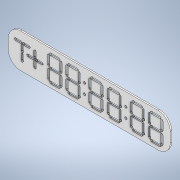
# Autodesk Inventor part: 7 Segment Clock
Saved by Autodesk Inventor 2021 (Build 250183000, 183)
## iProperties
Created: 2020-06-26
Part Number: 7 Segment Clock
Material: White
Document SubType Name: Modeling
Designer: dech3
Density: 1.188 g/cm^3
Appearance: Polycarbonate - Clear
Author: dech3
Autodesk Inventor part; units mm, degrees
(part 1 of 3)
ref_plane "YZ Plane" through (0, 0, 0) normal (1, 0, 0) x (0, 1, 0)
ref_plane "XZ Plane" through (0, 0, 0) normal (0, 1, 0) x (-1, 0, 0)
ref_plane "XY Plane" through (0, 0, 0) normal (0, 0, 1) x (1, 0, 0)
sketch "Single Segment" plane through (0, 0, 0) normal (0, 0, 1) x (1, 0, 0)
  arc A0 (128.9839, -2.0293) -> (129.691, -2.3222) centre (129.691, -1.3222) ccw
  arc A1 (129.691, 2.6778) -> (128.9839, 2.3849) centre (129.691, 1.6778) ccw
  line L0 (128.9839, -2.0293) -> (127.0768, -0.1222)
  line L1 (128.9839, 2.3849) -> (127.0768, 0.4778)
  line L2 (127.0768, 0.1778) -> (127.0768, -0.1222)
  line L3 (127.0768, 0.1778) -> (127.0768, 0.4778)
  line L4 (129.691, 2.6778) -> (146.4626, 2.6778)
  line L5 (146.4626, -2.3222) -> (129.691, -2.3222)
  arc A2 (147.1697, 2.3849) -> (146.4626, 2.6778) centre (146.4626, 1.6778) ccw
  line L6 (147.1697, 2.3849) -> (149.0768, 0.4778)
  line L7 (149.0768, 0.1778) -> (149.0768, 0.4778)
  line L8 (149.0768, 0.1778) -> (149.0768, -0.1222)
  arc A3 (146.4626, -2.3222) -> (147.1697, -2.0293) centre (146.4626, -1.3222) ccw
  line L9 (147.1697, -2.0293) -> (149.0768, -0.1222)
  point P0 (153.0768, 0)
  point P1 (129.2768, -2.3222)
  point P2 (129.2768, 2.6778)
  point P3 (146.8768, 2.6778)
  point P4 (146.8768, -2.3222)
  dimension "d105" = 2.2
  dimension "d108" = 2.2
  dimension "d111" = 2.2
  dimension "d112" = 2.2
  dimension "d113" = 2.2
  dimension "d114" = 2.2
  dimension "d115" = 2.2
  dimension "d116" = 1
  dimension "d117" = 5
  dimension "d121" = 2.2
  dimension "d122" = 2.2
  dimension "d126" = 135
  dimension "d127" = 22
  dimension "d128" = 135
  dimension "d129" = 2.5
  dimension "d348" = 5
  dimension "d349" = 22
  dimension "d350" = 2.2
  dimension "d352" = 0.3
  dimension "d353" = 0.3
  dimension "d358" = 0.3
  dimension "d359" = 0.3
  measures "d105" horizontal distance of point (129.277, -2.322) L0.end
  measures "d108" horizontal distance of L7.end point (146.877, 2.678)
  measures "d111" horizontal distance of point (129.277, 2.678) L3.end
  measures "d112" horizontal distance of L9.end point (146.877, -2.322)
  measures "d113" horizontal distance of L9.end point (146.877, -2.322)
  measures "d114" horizontal distance of point (129.277, 2.678) L3.end
  measures "d115" horizontal distance of point (129.277, -2.322) L0.end
  measures "d116" radius of A1
  measures "d117" distance of point (146.877, -2.322) point (146.877, 2.678)
  measures "d121" horizontal distance of L7.end point (146.877, 2.678)
  measures "d122" horizontal distance of point (146.877, -2.322) L8.start
  measures "d126" angle of L5 L9
  measures "d127" horizontal distance of L9.end L3.start
  measures "d128" angle of L4 L6
  measures "d129" vertical distance of L8.start point (146.877, -2.322)
  measures "d348" distance between parallel lines of L5 L4
  measures "d349" distance of L3.start L8.start
  measures "d350" horizontal distance of point (129.277, 2.678) L3.start
  measures "d352" distance of L8.start L7.end
  measures "d353" distance of L9.end L8.start
  measures "d358" distance of L3.end L3.start
  measures "d359" distance of L0.end L3.start
sketch "7 Segment Digit" plane through (0, 0, 0) normal (0, 0, 1) x (1, 0, 0)
  arc A0 (215.9071, -11.0293) -> (216.6142, -11.3222) centre (216.6142, -10.3222) ccw
  arc A1 (216.6142, -6.3222) -> (215.9071, -6.6151) centre (216.6142, -7.3222) ccw
  line L0 (215.9071, -11.0293) -> (214, -9.1222)
  line L1 (215.9071, -6.6151) -> (214, -8.5222)
  line L2 (214, -8.8222) -> (214, -9.1222)
  line L3 (214, -8.8222) -> (214, -8.5222)
  line L4 (216.6142, -6.3222) -> (233.3858, -6.3222)
  line L5 (233.3858, -11.3222) -> (216.6142, -11.3222)
  arc A2 (234.0929, -6.6151) -> (233.3858, -6.3222) centre (233.3858, -7.3222) ccw
  line L6 (234.0929, -6.6151) -> (236, -8.5222)
  line L7 (236, -8.8222) -> (236, -8.5222)
  line L8 (236, -8.8222) -> (236, -9.1222)
  arc A3 (233.3858, -11.3222) -> (234.0929, -11.0293) centre (233.3858, -10.3222) ccw
  line L9 (234.0929, -11.0293) -> (236, -9.1222)
  arc A4 (215.9071, -35.8293) -> (216.6142, -36.1222) centre (216.6142, -35.1222) ccw
  arc A5 (216.6142, -31.1222) -> (215.9071, -31.4151) centre (216.6142, -32.1222) ccw
  line L10 (215.9071, -35.8293) -> (214, -33.9222)
  line L11 (215.9071, -31.4151) -> (214, -33.3222)
  line L12 (214, -33.6222) -> (214, -33.9222)
  line L13 (214, -33.6222) -> (214, -33.3222)
  line L14 (216.6142, -31.1222) -> (233.3858, -31.1222)
  line L15 (233.3858, -36.1222) -> (216.6142, -36.1222)
  arc A6 (234.0929, -31.4151) -> (233.3858, -31.1222) centre (233.3858, -32.1222) ccw
  line L16 (234.0929, -31.4151) -> (236, -33.3222)
  line L17 (236, -33.6222) -> (236, -33.3222)
  line L18 (236, -33.6222) -> (236, -33.9222)
  arc A7 (233.3858, -36.1222) -> (234.0929, -35.8293) centre (233.3858, -35.1222) ccw
  line L19 (234.0929, -35.8293) -> (236, -33.9222)
  arc A8 (214.8071, -30.3151) -> (215.1, -29.608) centre (214.1, -29.608) ccw
  arc A9 (210.1, -29.608) -> (210.3929, -30.3151) centre (211.1, -29.608) ccw
  line L20 (214.8071, -30.3151) -> (212.9, -32.2222)
  line L21 (210.3929, -30.3151) -> (212.3, -32.2222)
  line L22 (212.6, -32.2222) -> (212.9, -32.2222)
  line L23 (212.6, -32.2222) -> (212.3, -32.2222)
  line L24 (210.1, -29.608) -> (210.1, -12.8364)
  line L25 (215.1, -12.8364) -> (215.1, -29.608)
  arc A10 (210.3929, -12.1293) -> (210.1, -12.8364) centre (211.1, -12.8364) ccw
  line L26 (210.3929, -12.1293) -> (212.3, -10.2222)
  line L27 (212.6, -10.2222) -> (212.3, -10.2222)
  line L28 (212.6, -10.2222) -> (212.9, -10.2222)
  arc A11 (215.1, -12.8364) -> (214.8071, -12.1293) centre (214.1, -12.8364) ccw
  line L29 (214.8071, -12.1293) -> (212.9, -10.2222)
  arc A12 (214.8071, -55.1151) -> (215.1, -54.408) centre (214.1, -54.408) ccw
  arc A13 (210.1, -54.408) -> (210.3929, -55.1151) centre (211.1, -54.408) ccw
  line L30 (214.8071, -55.1151) -> (212.9, -57.0222)
  line L31 (210.3929, -55.1151) -> (212.3, -57.0222)
  line L32 (212.6, -57.0222) -> (212.9, -57.0222)
  line L33 (212.6, -57.0222) -> (212.3, -57.0222)
  line L34 (210.1, -54.408) -> (210.1, -37.6364)
  line L35 (215.1, -37.6364) -> (215.1, -54.408)
  arc A14 (210.3929, -36.9293) -> (210.1, -37.6364) centre (211.1, -37.6364) ccw
  line L36 (210.3929, -36.9293) -> (212.3, -35.0222)
  line L37 (212.6, -35.0222) -> (212.3, -35.0222)
  line L38 (212.6, -35.0222) -> (212.9, -35.0222)
  arc A15 (215.1, -37.6364) -> (214.8071, -36.9293) centre (214.1, -37.6364) ccw
  line L39 (214.8071, -36.9293) -> (212.9, -35.0222)
  arc A16 (239.6071, -30.3151) -> (239.9, -29.608) centre (238.9, -29.608) ccw
  arc A17 (234.9, -29.608) -> (235.1929, -30.3151) centre (235.9, -29.608) ccw
  line L40 (239.6071, -30.3151) -> (237.7, -32.2222)
  line L41 (235.1929, -30.3151) -> (237.1, -32.2222)
  line L42 (237.4, -32.2222) -> (237.7, -32.2222)
  line L43 (237.4, -32.2222) -> (237.1, -32.2222)
  line L44 (234.9, -29.608) -> (234.9, -12.8364)
  line L45 (239.9, -12.8364) -> (239.9, -29.608)
  arc A18 (235.1929, -12.1293) -> (234.9, -12.8364) centre (235.9, -12.8364) ccw
  line L46 (235.1929, -12.1293) -> (237.1, -10.2222)
  line L47 (237.4, -10.2222) -> (237.1, -10.2222)
  line L48 (237.4, -10.2222) -> (237.7, -10.2222)
  arc A19 (239.9, -12.8364) -> (239.6071, -12.1293) centre (238.9, -12.8364) ccw
  line L49 (239.6071, -12.1293) -> (237.7, -10.2222)
  arc A20 (239.6071, -55.1151) -> (239.9, -54.408) centre (238.9, -54.408) ccw
  arc A21 (234.9, -54.408) -> (235.1929, -55.1151) centre (235.9, -54.408) ccw
  line L50 (239.6071, -55.1151) -> (237.7, -57.0222)
  line L51 (235.1929, -55.1151) -> (237.1, -57.0222)
  line L52 (237.4, -57.0222) -> (237.7, -57.0222)
  line L53 (237.4, -57.0222) -> (237.1, -57.0222)
  line L54 (234.9, -54.408) -> (234.9, -37.6364)
  line L55 (239.9, -37.6364) -> (239.9, -54.408)
  arc A22 (235.1929, -36.9293) -> (234.9, -37.6364) centre (235.9, -37.6364) ccw
  line L56 (235.1929, -36.9293) -> (237.1, -35.0222)
  line L57 (237.4, -35.0222) -> (237.1, -35.0222)
  line L58 (237.4, -35.0222) -> (237.7, -35.0222)
  arc A23 (239.9, -37.6364) -> (239.6071, -36.9293) centre (238.9, -37.6364) ccw
  line L59 (239.6071, -36.9293) -> (237.7, -35.0222)
  arc A24 (215.9071, -60.6293) -> (216.6142, -60.9222) centre (216.6142, -59.9222) ccw
  arc A25 (216.6142, -55.9222) -> (215.9071, -56.2151) centre (216.6142, -56.9222) ccw
  line L60 (215.9071, -60.6293) -> (214, -58.7222)
  line L61 (215.9071, -56.2151) -> (214, -58.1222)
  line L62 (214, -58.4222) -> (214, -58.7222)
  line L63 (214, -58.4222) -> (214, -58.1222)
  line L64 (216.6142, -55.9222) -> (233.3858, -55.9222)
  line L65 (233.3858, -60.9222) -> (216.6142, -60.9222)
  arc A26 (234.0929, -56.2151) -> (233.3858, -55.9222) centre (233.3858, -56.9222) ccw
  line L66 (234.0929, -56.2151) -> (236, -58.1222)
  line L67 (236, -58.4222) -> (236, -58.1222)
  line L68 (236, -58.4222) -> (236, -58.7222)
  arc A27 (233.3858, -60.9222) -> (234.0929, -60.6293) centre (233.3858, -59.9222) ccw
  line L69 (234.0929, -60.6293) -> (236, -58.7222)
  point P0 (239.8857, -4.9143)
  dimension "d131" = 1.1
  dimension "d132" = 1.1
  dimension "d137" = 1.1
  dimension "d138" = 1.1
  dimension "d139" = 1.1
  dimension "d140" = 1.1
  dimension "d141" = 1.1
  dimension "d142" = 1.1
  dimension "d143" = 1.1
  dimension "d144" = 1.1
  dimension "d145" = 1.1
  dimension "d146" = 1.1
  dimension "d150" = 1.1
  dimension "d151" = 1.1
  dimension "d152" = 1.1
  dimension "d153" = 1.1
sketch "Slanted Segment Large" plane through (0, 0, 0) normal (0, 0, 1) x (1, 0, 0)
  line L0 (-252.8296, -124.6537) -> (-254.4296, -124.6537)
  line L1 (-254.4296, -124.6537) -> (-257.6296, -127.8537)
  line L2 (-257.6296, -127.8537) -> (-261.6917, -184.8537)
  line L3 (-253.6917, -184.8537) -> (-249.6296, -127.8537)
  line L4 (-249.6296, -127.8537) -> (-252.8296, -124.6537)
  line L5 (-261.6917, -184.8537) -> (-258.4917, -188.0537)
  line L6 (-258.4917, -188.0537) -> (-256.8917, -188.0537)
  line L7 (-256.8917, -188.0537) -> (-253.6917, -184.8537)
  point P0 (-253.3255, -154.094)
  point P1 (-253.6296, -124.6537)
  dimension "d294" = 3.2
  dimension "d295" = 3.2
  dimension "d296" = 8
  dimension "d297" = 3.2
  dimension "d298" = 3.2
  dimension "d299" = 57
  dimension "d304" = 3.2
  dimension "d305" = 3.2
  dimension "d306" = 3.2
  dimension "d307" = 3.2
  measures "d294" horizontal distance of L0.end L1.end
  measures "d295" horizontal distance of L3.end L0.start
  measures "d296" distance of L3.end L1.end
  measures "d297" horizontal distance of L3.end L0.start
  measures "d298" horizontal distance of L0.end L1.end
  measures "d299" vertical distance of L3.end L3.start
  measures "d304" horizontal distance of L5.end L2.end
  measures "d305" horizontal distance of L3.start L6.end
  measures "d306" horizontal distance of L2.end L5.end
  measures "d307" horizontal distance of L3.start L6.end
sketch "+ sign" plane through (0, 0, 0) normal (0, 0, 1) x (1, 0, 0)
  arc A0 (1.761, -2.8041) -> (2.4681, -3.097) centre (2.4681, -2.097) ccw
  arc A1 (2.4681, 1.903) -> (1.761, 1.6102) centre (2.4681, 0.903) ccw
  line L0 (1.761, -2.8041) -> (-0.1461, -0.897)
  line L1 (-0.1461, -0.597) -> (-0.1461, -0.297)
  line L2 (-0.1461, -0.597) -> (-0.1461, -0.897)
  line L3 (1.761, 1.6102) -> (-0.1461, -0.297)
  line L4 (2.4681, 1.903) -> (13.2397, 1.903)
  line L5 (13.2397, -3.097) -> (2.4681, -3.097)
  arc A2 (13.9468, 1.6102) -> (13.2397, 1.903) centre (13.2397, 0.903) ccw
  arc A3 (13.2397, -3.097) -> (13.9468, -2.8041) centre (13.2397, -2.097) ccw
  line L6 (13.9468, -2.8041) -> (15.8539, -0.897)
  line L7 (15.8539, -0.597) -> (15.8539, -0.897)
  line L8 (15.8539, -0.597) -> (15.8539, -0.297)
  line L9 (13.9468, 1.6102) -> (15.8539, -0.297)
  arc A4 (1.061, 2.3102) -> (1.3539, 3.0173) centre (0.3539, 3.0173) ccw
  arc A5 (-3.6461, 3.0173) -> (-3.3532, 2.3102) centre (-2.6461, 3.0173) ccw
  line L10 (1.061, 2.3102) -> (-0.8461, 0.403)
  line L11 (-1.1461, 0.403) -> (-1.4461, 0.403)
  line L12 (-1.1461, 0.403) -> (-0.8461, 0.403)
  line L13 (-3.3532, 2.3102) -> (-1.4461, 0.403)
  line L14 (-3.6461, 3.0173) -> (-3.6461, 13.7888)
  line L15 (1.3539, 13.7888) -> (1.3539, 3.0173)
  arc A6 (-3.3532, 14.4959) -> (-3.6461, 13.7888) centre (-2.6461, 13.7888) ccw
  arc A7 (1.3539, 13.7888) -> (1.061, 14.4959) centre (0.3539, 13.7888) ccw
  line L16 (1.061, 14.4959) -> (-0.8461, 16.403)
  line L17 (-1.1461, 16.403) -> (-0.8461, 16.403)
  line L18 (-1.1461, 16.403) -> (-1.4461, 16.403)
  line L19 (-3.3532, 14.4959) -> (-1.4461, 16.403)
  arc A8 (-16.239, -2.8041) -> (-15.5319, -3.097) centre (-15.5319, -2.097) ccw
  arc A9 (-15.5319, 1.903) -> (-16.239, 1.6102) centre (-15.5319, 0.903) ccw
  line L20 (-16.239, -2.8041) -> (-18.1461, -0.897)
  line L21 (-18.1461, -0.597) -> (-18.1461, -0.297)
  line L22 (-18.1461, -0.597) -> (-18.1461, -0.897)
  line L23 (-16.239, 1.6102) -> (-18.1461, -0.297)
  line L24 (-15.5319, 1.903) -> (-4.7603, 1.903)
  line L25 (-4.7603, -3.097) -> (-15.5319, -3.097)
  arc A10 (-4.0532, 1.6102) -> (-4.7603, 1.903) centre (-4.7603, 0.903) ccw
  arc A11 (-4.7603, -3.097) -> (-4.0532, -2.8041) centre (-4.7603, -2.097) ccw
  line L26 (-4.0532, -2.8041) -> (-2.1461, -0.897)
  line L27 (-2.1461, -0.597) -> (-2.1461, -0.897)
  line L28 (-2.1461, -0.597) -> (-2.1461, -0.297)
  line L29 (-4.0532, 1.6102) -> (-2.1461, -0.297)
  arc A12 (1.061, -15.6898) -> (1.3539, -14.9827) centre (0.3539, -14.9827) ccw
  arc A13 (-3.6461, -14.9827) -> (-3.3532, -15.6898) centre (-2.6461, -14.9827) ccw
  line L30 (1.061, -15.6898) -> (-0.8461, -17.597)
  line L31 (-1.1461, -17.597) -> (-1.4461, -17.597)
  line L32 (-1.1461, -17.597) -> (-0.8461, -17.597)
  line L33 (-3.3532, -15.6898) -> (-1.4461, -17.597)
  line L34 (-3.6461, -14.9827) -> (-3.6461, -4.2112)
  line L35 (1.3539, -4.2112) -> (1.3539, -14.9827)
  arc A14 (-3.3532, -3.5041) -> (-3.6461, -4.2112) centre (-2.6461, -4.2112) ccw
  arc A15 (1.3539, -4.2112) -> (1.061, -3.5041) centre (0.3539, -4.2112) ccw
  line L36 (1.061, -3.5041) -> (-0.8461, -1.597)
  line L37 (-1.1461, -1.597) -> (-0.8461, -1.597)
  line L38 (-1.1461, -1.597) -> (-1.4461, -1.597)
  line L39 (-3.3532, -3.5041) -> (-1.4461, -1.597)
  point P0 (-225.4266, -6.7349)
  dimension "d496" = 2
  dimension "d497" = 2
  dimension "d501" = 1
  dimension "d502" = 1
  dimension "d503" = 0
  dimension "d504" = 0
  dimension "d505" = 0.99
  dimension "d506" = 0.99
  dimension "d507" = 0.99
  dimension "d508" = 0.99
sketch "Dot" plane through (0, 0, 0) normal (0, 0, 1) x (1, 0, 0)
  line L0 (-36.1663, 28.3091) -> (-35.1663, 28.3091)
  line L1 (-35.1663, 28.3091) -> (-33.1663, 26.3091)
  line L2 (-33.1663, 26.3091) -> (-33.1663, 25.3091)
  line L3 (-33.1663, 25.3091) -> (-35.1663, 23.3091)
  line L4 (-35.1663, 23.3091) -> (-36.1663, 23.3091)
  line L5 (-36.1663, 23.3091) -> (-38.1663, 25.3091)
  line L6 (-38.1663, 25.3091) -> (-38.1663, 26.3091)
  line L7 (-38.1663, 26.3091) -> (-36.1663, 28.3091)
  point P0 (-33.9663, 25.3091)
  dimension "d311" = 2
  dimension "d312" = 2
  dimension "d314" = 2
  dimension "d315" = 2
  dimension "d316" = 2
  dimension "d317" = 2
  dimension "d318" = 2
  dimension "d319" = 2
  dimension "d320" = 1
  dimension "d321" = 1
  dimension "d322" = 1
  dimension "d323" = 1
  dimension "d360" = 5
  dimension "d361" = 5
  measures "d311" horizontal distance of L1.end L0.end
  measures "d312" horizontal distance of L0.start L6.end
  measures "d314" horizontal distance of L0.start L6.end
  measures "d315" horizontal distance of L1.end L0.end
  measures "d316" horizontal distance of L4.end L5.end
  measures "d317" horizontal distance of L2.end L3.end
  measures "d318" horizontal distance of L2.end L3.end
  measures "d319" horizontal distance of L5.end L4.end
  measures "d320" distance of L1.end L2.end
  measures "d321" distance of L0.end L0.start
  measures "d322" distance of L3.end L4.end
  measures "d323" distance of L6.end L5.end
  measures "d360" distance between parallel lines of L4 L0
  measures "d361" distance between parallel lines of L2 L6
sketch "Clock Face with T +-" plane through (0, 0, 0) normal (0, 0, 1) x (1, 0, 0)
  arc A0 (53.0672, 19.3353) -> (53.7743, 19.0424) centre (53.7743, 20.0424) ccw
  arc A1 (53.7743, 24.0424) -> (53.0672, 23.7495) centre (53.7743, 23.0424) ccw
  line L0 (53.0672, 19.3353) -> (51.1601, 21.2424)
  line L1 (53.0672, 23.7495) -> (51.1601, 21.8424)
  line L2 (51.1601, 21.5424) -> (51.1601, 21.2424)
  line L3 (51.1601, 21.5424) -> (51.1601, 21.8424)
  line L4 (53.7743, 24.0424) -> (70.5459, 24.0424)
  line L5 (70.5459, 19.0424) -> (53.7743, 19.0424)
  arc A2 (71.253, 23.7495) -> (70.5459, 24.0424) centre (70.5459, 23.0424) ccw
  line L6 (71.253, 23.7495) -> (73.1601, 21.8424)
  line L7 (73.1601, 21.5424) -> (73.1601, 21.8424)
  line L8 (73.1601, 21.5424) -> (73.1601, 21.2424)
  arc A3 (70.5459, 19.0424) -> (71.253, 19.3353) centre (70.5459, 20.0424) ccw
  line L9 (71.253, 19.3353) -> (73.1601, 21.2424)
  arc A4 (53.0672, -5.4647) -> (53.7743, -5.7576) centre (53.7743, -4.7576) ccw
  arc A5 (53.7743, -0.7576) -> (53.0672, -1.0505) centre (53.7743, -1.7576) ccw
  line L10 (53.0672, -5.4647) -> (51.1601, -3.5576)
  line L11 (53.0672, -1.0505) -> (51.1601, -2.9576)
  line L12 (51.1601, -3.2576) -> (51.1601, -3.5576)
  line L13 (51.1601, -3.2576) -> (51.1601, -2.9576)
  line L14 (53.7743, -0.7576) -> (70.5459, -0.7576)
  line L15 (70.5459, -5.7576) -> (53.7743, -5.7576)
  arc A6 (71.253, -1.0505) -> (70.5459, -0.7576) centre (70.5459, -1.7576) ccw
  line L16 (71.253, -1.0505) -> (73.1601, -2.9576)
  line L17 (73.1601, -3.2576) -> (73.1601, -2.9576)
  line L18 (73.1601, -3.2576) -> (73.1601, -3.5576)
  arc A7 (70.5459, -5.7576) -> (71.253, -5.4647) centre (70.5459, -4.7576) ccw
  line L19 (71.253, -5.4647) -> (73.1601, -3.5576)
  arc A8 (51.9672, 0.0495) -> (52.2601, 0.7566) centre (51.2601, 0.7566) ccw
  arc A9 (47.2601, 0.7566) -> (47.553, 0.0495) centre (48.2601, 0.7566) ccw
  line L20 (51.9672, 0.0495) -> (50.0601, -1.8576)
  line L21 (47.553, 0.0495) -> (49.4601, -1.8576)
  line L22 (49.7601, -1.8576) -> (50.0601, -1.8576)
  line L23 (49.7601, -1.8576) -> (49.4601, -1.8576)
  line L24 (47.2601, 0.7566) -> (47.2601, 17.5282)
  line L25 (52.2601, 17.5282) -> (52.2601, 0.7566)
  arc A10 (47.553, 18.2353) -> (47.2601, 17.5282) centre (48.2601, 17.5282) ccw
  line L26 (47.553, 18.2353) -> (49.4601, 20.1424)
  line L27 (49.7601, 20.1424) -> (49.4601, 20.1424)
  line L28 (49.7601, 20.1424) -> (50.0601, 20.1424)
  arc A11 (52.2601, 17.5282) -> (51.9672, 18.2353) centre (51.2601, 17.5282) ccw
  line L29 (51.9672, 18.2353) -> (50.0601, 20.1424)
  arc A12 (51.9672, -24.7505) -> (52.2601, -24.0434) centre (51.2601, -24.0434) ccw
  arc A13 (47.2601, -24.0434) -> (47.553, -24.7505) centre (48.2601, -24.0434) ccw
  line L30 (51.9672, -24.7505) -> (50.0601, -26.6576)
  line L31 (47.553, -24.7505) -> (49.4601, -26.6576)
  line L32 (49.7601, -26.6576) -> (50.0601, -26.6576)
  line L33 (49.7601, -26.6576) -> (49.4601, -26.6576)
  line L34 (47.2601, -24.0434) -> (47.2601, -7.2718)
  line L35 (52.2601, -7.2718) -> (52.2601, -24.0434)
  arc A14 (47.553, -6.5647) -> (47.2601, -7.2718) centre (48.2601, -7.2718) ccw
  line L36 (47.553, -6.5647) -> (49.4601, -4.6576)
  line L37 (49.7601, -4.6576) -> (49.4601, -4.6576)
  line L38 (49.7601, -4.6576) -> (50.0601, -4.6576)
  arc A15 (52.2601, -7.2718) -> (51.9672, -6.5647) centre (51.2601, -7.2718) ccw
  line L39 (51.9672, -6.5647) -> (50.0601, -4.6576)
  arc A16 (76.7672, 0.0495) -> (77.0601, 0.7566) centre (76.0601, 0.7566) ccw
  arc A17 (72.0601, 0.7566) -> (72.353, 0.0495) centre (73.0601, 0.7566) ccw
  line L40 (76.7672, 0.0495) -> (74.8601, -1.8576)
  line L41 (72.353, 0.0495) -> (74.2601, -1.8576)
  line L42 (74.5601, -1.8576) -> (74.8601, -1.8576)
  line L43 (74.5601, -1.8576) -> (74.2601, -1.8576)
  line L44 (72.0601, 0.7566) -> (72.0601, 17.5282)
  line L45 (77.0601, 17.5282) -> (77.0601, 0.7566)
  arc A18 (72.353, 18.2353) -> (72.0601, 17.5282) centre (73.0601, 17.5282) ccw
  line L46 (72.353, 18.2353) -> (74.2601, 20.1424)
  line L47 (74.5601, 20.1424) -> (74.2601, 20.1424)
  line L48 (74.5601, 20.1424) -> (74.8601, 20.1424)
  arc A19 (77.0601, 17.5282) -> (76.7672, 18.2353) centre (76.0601, 17.5282) ccw
  line L49 (76.7672, 18.2353) -> (74.8601, 20.1424)
  arc A20 (76.7672, -24.7505) -> (77.0601, -24.0434) centre (76.0601, -24.0434) ccw
  arc A21 (72.0601, -24.0434) -> (72.353, -24.7505) centre (73.0601, -24.0434) ccw
  line L50 (76.7672, -24.7505) -> (74.8601, -26.6576)
  line L51 (72.353, -24.7505) -> (74.2601, -26.6576)
  line L52 (74.5601, -26.6576) -> (74.8601, -26.6576)
  line L53 (74.5601, -26.6576) -> (74.2601, -26.6576)
  line L54 (72.0601, -24.0434) -> (72.0601, -7.2718)
  line L55 (77.0601, -7.2718) -> (77.0601, -24.0434)
  arc A22 (72.353, -6.5647) -> (72.0601, -7.2718) centre (73.0601, -7.2718) ccw
  line L56 (72.353, -6.5647) -> (74.2601, -4.6576)
  line L57 (74.5601, -4.6576) -> (74.2601, -4.6576)
  line L58 (74.5601, -4.6576) -> (74.8601, -4.6576)
  arc A23 (77.0601, -7.2718) -> (76.7672, -6.5647) centre (76.0601, -7.2718) ccw
  line L59 (76.7672, -6.5647) -> (74.8601, -4.6576)
  arc A24 (53.0672, -30.2647) -> (53.7743, -30.5576) centre (53.7743, -29.5576) ccw
  arc A25 (53.7743, -25.5576) -> (53.0672, -25.8505) centre (53.7743, -26.5576) ccw
  line L60 (53.0672, -30.2647) -> (51.1601, -28.3576)
  line L61 (53.0672, -25.8505) -> (51.1601, -27.7576)
  line L62 (51.1601, -28.0576) -> (51.1601, -28.3576)
  line L63 (51.1601, -28.0576) -> (51.1601, -27.7576)
  line L64 (53.7743, -25.5576) -> (70.5459, -25.5576)
  line L65 (70.5459, -30.5576) -> (53.7743, -30.5576)
  arc A26 (71.253, -25.8505) -> (70.5459, -25.5576) centre (70.5459, -26.5576) ccw
  line L66 (71.253, -25.8505) -> (73.1601, -27.7576)
  line L67 (73.1601, -28.0576) -> (73.1601, -27.7576)
  line L68 (73.1601, -28.0576) -> (73.1601, -28.3576)
  arc A27 (70.5459, -30.5576) -> (71.253, -30.2647) centre (70.5459, -29.5576) ccw
  line L69 (71.253, -30.2647) -> (73.1601, -28.3576)
  arc A28 (6.2672, 19.3353) -> (6.9743, 19.0424) centre (6.9743, 20.0424) ccw
  arc A29 (6.9743, 24.0424) -> (6.2672, 23.7495) centre (6.9743, 23.0424) ccw
  line L70 (6.2672, 19.3353) -> (4.3601, 21.2424)
  line L71 (6.2672, 23.7495) -> (4.3601, 21.8424)
  line L72 (4.3601, 21.5424) -> (4.3601, 21.2424)
  line L73 (4.3601, 21.5424) -> (4.3601, 21.8424)
  line L74 (6.9743, 24.0424) -> (23.7459, 24.0424)
  line L75 (23.7459, 19.0424) -> (6.9743, 19.0424)
  arc A30 (24.453, 23.7495) -> (23.7459, 24.0424) centre (23.7459, 23.0424) ccw
  line L76 (24.453, 23.7495) -> (26.3601, 21.8424)
  line L77 (26.3601, 21.5424) -> (26.3601, 21.8424)
  line L78 (26.3601, 21.5424) -> (26.3601, 21.2424)
  arc A31 (23.7459, 19.0424) -> (24.453, 19.3353) centre (23.7459, 20.0424) ccw
  line L79 (24.453, 19.3353) -> (26.3601, 21.2424)
  arc A32 (6.2672, -5.4647) -> (6.9743, -5.7576) centre (6.9743, -4.7576) ccw
  arc A33 (6.9743, -0.7576) -> (6.2672, -1.0505) centre (6.9743, -1.7576) ccw
  line L80 (6.2672, -5.4647) -> (4.3601, -3.5576)
  line L81 (6.2672, -1.0505) -> (4.3601, -2.9576)
  line L82 (4.3601, -3.2576) -> (4.3601, -3.5576)
  line L83 (4.3601, -3.2576) -> (4.3601, -2.9576)
  line L84 (6.9743, -0.7576) -> (23.7459, -0.7576)
  line L85 (23.7459, -5.7576) -> (6.9743, -5.7576)
  arc A34 (24.453, -1.0505) -> (23.7459, -0.7576) centre (23.7459, -1.7576) ccw
  line L86 (24.453, -1.0505) -> (26.3601, -2.9576)
  line L87 (26.3601, -3.2576) -> (26.3601, -2.9576)
  line L88 (26.3601, -3.2576) -> (26.3601, -3.5576)
  arc A35 (23.7459, -5.7576) -> (24.453, -5.4647) centre (23.7459, -4.7576) ccw
  line L89 (24.453, -5.4647) -> (26.3601, -3.5576)
  arc A36 (5.1672, 0.0495) -> (5.4601, 0.7566) centre (4.4601, 0.7566) ccw
  arc A37 (0.4601, 0.7566) -> (0.753, 0.0495) centre (1.4601, 0.7566) ccw
  line L90 (5.1672, 0.0495) -> (3.2601, -1.8576)
  line L91 (0.753, 0.0495) -> (2.6601, -1.8576)
  line L92 (2.9601, -1.8576) -> (3.2601, -1.8576)
  line L93 (2.9601, -1.8576) -> (2.6601, -1.8576)
  line L94 (0.4601, 0.7566) -> (0.4601, 17.5282)
  line L95 (5.4601, 17.5282) -> (5.4601, 0.7566)
  arc A38 (0.753, 18.2353) -> (0.4601, 17.5282) centre (1.4601, 17.5282) ccw
  line L96 (0.753, 18.2353) -> (2.6601, 20.1424)
  line L97 (2.9601, 20.1424) -> (2.6601, 20.1424)
  line L98 (2.9601, 20.1424) -> (3.2601, 20.1424)
  arc A39 (5.4601, 17.5282) -> (5.1672, 18.2353) centre (4.4601, 17.5282) ccw
  line L99 (5.1672, 18.2353) -> (3.2601, 20.1424)
  arc A40 (5.1672, -24.7505) -> (5.4601, -24.0434) centre (4.4601, -24.0434) ccw
  arc A41 (0.4601, -24.0434) -> (0.753, -24.7505) centre (1.4601, -24.0434) ccw
  line L100 (5.1672, -24.7505) -> (3.2601, -26.6576)
  line L101 (0.753, -24.7505) -> (2.6601, -26.6576)
  line L102 (2.9601, -26.6576) -> (3.2601, -26.6576)
  line L103 (2.9601, -26.6576) -> (2.6601, -26.6576)
  line L104 (0.4601, -24.0434) -> (0.4601, -7.2718)
  line L105 (5.4601, -7.2718) -> (5.4601, -24.0434)
  arc A42 (0.753, -6.5647) -> (0.4601, -7.2718) centre (1.4601, -7.2718) ccw
  line L106 (0.753, -6.5647) -> (2.6601, -4.6576)
  line L107 (2.9601, -4.6576) -> (2.6601, -4.6576)
  line L108 (2.9601, -4.6576) -> (3.2601, -4.6576)
  arc A43 (5.4601, -7.2718) -> (5.1672, -6.5647) centre (4.4601, -7.2718) ccw
  line L109 (5.1672, -6.5647) -> (3.2601, -4.6576)
  arc A44 (29.9672, 0.0495) -> (30.2601, 0.7566) centre (29.2601, 0.7566) ccw
  arc A45 (25.2601, 0.7566) -> (25.553, 0.0495) centre (26.2601, 0.7566) ccw
  line L110 (29.9672, 0.0495) -> (28.0601, -1.8576)
  line L111 (25.553, 0.0495) -> (27.4601, -1.8576)
  line L112 (27.7601, -1.8576) -> (28.0601, -1.8576)
  line L113 (27.7601, -1.8576) -> (27.4601, -1.8576)
  line L114 (25.2601, 0.7566) -> (25.2601, 17.5282)
  line L115 (30.2601, 17.5282) -> (30.2601, 0.7566)
  arc A46 (25.553, 18.2353) -> (25.2601, 17.5282) centre (26.2601, 17.5282) ccw
  line L116 (25.553, 18.2353) -> (27.4601, 20.1424)
  line L117 (27.7601, 20.1424) -> (27.4601, 20.1424)
  line L118 (27.7601, 20.1424) -> (28.0601, 20.1424)
  arc A47 (30.2601, 17.5282) -> (29.9672, 18.2353) centre (29.2601, 17.5282) ccw
  line L119 (29.9672, 18.2353) -> (28.0601, 20.1424)
  arc A48 (29.9672, -24.7505) -> (30.2601, -24.0434) centre (29.2601, -24.0434) ccw
  arc A49 (25.2601, -24.0434) -> (25.553, -24.7505) centre (26.2601, -24.0434) ccw
  line L120 (29.9672, -24.7505) -> (28.0601, -26.6576)
  line L121 (25.553, -24.7505) -> (27.4601, -26.6576)
  line L122 (27.7601, -26.6576) -> (28.0601, -26.6576)
  line L123 (27.7601, -26.6576) -> (27.4601, -26.6576)
  line L124 (25.2601, -24.0434) -> (25.2601, -7.2718)
  line L125 (30.2601, -7.2718) -> (30.2601, -24.0434)
  arc A50 (25.553, -6.5647) -> (25.2601, -7.2718) centre (26.2601, -7.2718) ccw
  line L126 (25.553, -6.5647) -> (27.4601, -4.6576)
  line L127 (27.7601, -4.6576) -> (27.4601, -4.6576)
  line L128 (27.7601, -4.6576) -> (28.0601, -4.6576)
  arc A51 (30.2601, -7.2718) -> (29.9672, -6.5647) centre (29.2601, -7.2718) ccw
  line L129 (29.9672, -6.5647) -> (28.0601, -4.6576)
  arc A52 (6.2672, -30.2647) -> (6.9743, -30.5576) centre (6.9743, -29.5576) ccw
  arc A53 (6.9743, -25.5576) -> (6.2672, -25.8505) centre (6.9743, -26.5576) ccw
  line L130 (6.2672, -30.2647) -> (4.3601, -28.3576)
  line L131 (6.2672, -25.8505) -> (4.3601, -27.7576)
  line L132 (4.3601, -28.0576) -> (4.3601, -28.3576)
  line L133 (4.3601, -28.0576) -> (4.3601, -27.7576)
  line L134 (6.9743, -25.5576) -> (23.7459, -25.5576)
  line L135 (23.7459, -30.5576) -> (6.9743, -30.5576)
  arc A54 (24.453, -25.8505) -> (23.7459, -25.5576) centre (23.7459, -26.5576) ccw
  line L136 (24.453, -25.8505) -> (26.3601, -27.7576)
  line L137 (26.3601, -28.0576) -> (26.3601, -27.7576)
  line L138 (26.3601, -28.0576) -> (26.3601, -28.3576)
  arc A55 (23.7459, -30.5576) -> (24.453, -30.2647) centre (23.7459, -29.5576) ccw
  line L139 (24.453, -30.2647) -> (26.3601, -28.3576)
  arc A56 (-31.0328, 19.3353) -> (-30.3257, 19.0424) centre (-30.3257, 20.0424) ccw
  arc A57 (-30.3257, 24.0424) -> (-31.0328, 23.7495) centre (-30.3257, 23.0424) ccw
  line L140 (-31.0328, 19.3353) -> (-32.9399, 21.2424)
  line L141 (-31.0328, 23.7495) -> (-32.9399, 21.8424)
  line L142 (-32.9399, 21.5424) -> (-32.9399, 21.2424)
  line L143 (-32.9399, 21.5424) -> (-32.9399, 21.8424)
  line L144 (-30.3257, 24.0424) -> (-13.5541, 24.0424)
  line L145 (-13.5541, 19.0424) -> (-30.3257, 19.0424)
  arc A58 (-12.847, 23.7495) -> (-13.5541, 24.0424) centre (-13.5541, 23.0424) ccw
  line L146 (-12.847, 23.7495) -> (-10.9399, 21.8424)
  line L147 (-10.9399, 21.5424) -> (-10.9399, 21.8424)
  line L148 (-10.9399, 21.5424) -> (-10.9399, 21.2424)
  arc A59 (-13.5541, 19.0424) -> (-12.847, 19.3353) centre (-13.5541, 20.0424) ccw
  line L149 (-12.847, 19.3353) -> (-10.9399, 21.2424)
  arc A60 (-31.0328, -5.4647) -> (-30.3257, -5.7576) centre (-30.3257, -4.7576) ccw
  arc A61 (-30.3257, -0.7576) -> (-31.0328, -1.0505) centre (-30.3257, -1.7576) ccw
  line L150 (-31.0328, -5.4647) -> (-32.9399, -3.5576)
  line L151 (-31.0328, -1.0505) -> (-32.9399, -2.9576)
  line L152 (-32.9399, -3.2576) -> (-32.9399, -3.5576)
  line L153 (-32.9399, -3.2576) -> (-32.9399, -2.9576)
  line L154 (-30.3257, -0.7576) -> (-13.5541, -0.7576)
  line L155 (-13.5541, -5.7576) -> (-30.3257, -5.7576)
  arc A62 (-12.847, -1.0505) -> (-13.5541, -0.7576) centre (-13.5541, -1.7576) ccw
  line L156 (-12.847, -1.0505) -> (-10.9399, -2.9576)
  line L157 (-10.9399, -3.2576) -> (-10.9399, -2.9576)
  line L158 (-10.9399, -3.2576) -> (-10.9399, -3.5576)
  arc A63 (-13.5541, -5.7576) -> (-12.847, -5.4647) centre (-13.5541, -4.7576) ccw
  line L159 (-12.847, -5.4647) -> (-10.9399, -3.5576)
  arc A64 (-32.1328, 0.0495) -> (-31.8399, 0.7566) centre (-32.8399, 0.7566) ccw
  arc A65 (-36.8399, 0.7566) -> (-36.547, 0.0495) centre (-35.8399, 0.7566) ccw
  line L160 (-32.1328, 0.0495) -> (-34.0399, -1.8576)
  line L161 (-36.547, 0.0495) -> (-34.6399, -1.8576)
  line L162 (-34.3399, -1.8576) -> (-34.0399, -1.8576)
  line L163 (-34.3399, -1.8576) -> (-34.6399, -1.8576)
  line L164 (-36.8399, 0.7566) -> (-36.8399, 17.5282)
  line L165 (-31.8399, 17.5282) -> (-31.8399, 0.7566)
  arc A66 (-36.547, 18.2353) -> (-36.8399, 17.5282) centre (-35.8399, 17.5282) ccw
  line L166 (-36.547, 18.2353) -> (-34.6399, 20.1424)
  line L167 (-34.3399, 20.1424) -> (-34.6399, 20.1424)
  line L168 (-34.3399, 20.1424) -> (-34.0399, 20.1424)
  arc A67 (-31.8399, 17.5282) -> (-32.1328, 18.2353) centre (-32.8399, 17.5282) ccw
  line L169 (-32.1328, 18.2353) -> (-34.0399, 20.1424)
  arc A68 (-32.1328, -24.7505) -> (-31.8399, -24.0434) centre (-32.8399, -24.0434) ccw
  arc A69 (-36.8399, -24.0434) -> (-36.547, -24.7505) centre (-35.8399, -24.0434) ccw
  line L170 (-32.1328, -24.7505) -> (-34.0399, -26.6576)
  line L171 (-36.547, -24.7505) -> (-34.6399, -26.6576)
  line L172 (-34.3399, -26.6576) -> (-34.0399, -26.6576)
  line L173 (-34.3399, -26.6576) -> (-34.6399, -26.6576)
  line L174 (-36.8399, -24.0434) -> (-36.8399, -7.2718)
  line L175 (-31.8399, -7.2718) -> (-31.8399, -24.0434)
  arc A70 (-36.547, -6.5647) -> (-36.8399, -7.2718) centre (-35.8399, -7.2718) ccw
  line L176 (-36.547, -6.5647) -> (-34.6399, -4.6576)
  line L177 (-34.3399, -4.6576) -> (-34.6399, -4.6576)
  line L178 (-34.3399, -4.6576) -> (-34.0399, -4.6576)
  arc A71 (-31.8399, -7.2718) -> (-32.1328, -6.5647) centre (-32.8399, -7.2718) ccw
  line L179 (-32.1328, -6.5647) -> (-34.0399, -4.6576)
  arc A72 (-7.3328, 0.0495) -> (-7.0399, 0.7566) centre (-8.0399, 0.7566) ccw
  arc A73 (-12.0399, 0.7566) -> (-11.747, 0.0495) centre (-11.0399, 0.7566) ccw
  line L180 (-7.3328, 0.0495) -> (-9.2399, -1.8576)
  line L181 (-11.747, 0.0495) -> (-9.8399, -1.8576)
  line L182 (-9.5399, -1.8576) -> (-9.2399, -1.8576)
  line L183 (-9.5399, -1.8576) -> (-9.8399, -1.8576)
  line L184 (-12.0399, 0.7566) -> (-12.0399, 17.5282)
  line L185 (-7.0399, 17.5282) -> (-7.0399, 0.7566)
  arc A74 (-11.747, 18.2353) -> (-12.0399, 17.5282) centre (-11.0399, 17.5282) ccw
  line L186 (-11.747, 18.2353) -> (-9.8399, 20.1424)
  line L187 (-9.5399, 20.1424) -> (-9.8399, 20.1424)
  line L188 (-9.5399, 20.1424) -> (-9.2399, 20.1424)
  arc A75 (-7.0399, 17.5282) -> (-7.3328, 18.2353) centre (-8.0399, 17.5282) ccw
  line L189 (-7.3328, 18.2353) -> (-9.2399, 20.1424)
  arc A76 (-7.3328, -24.7505) -> (-7.0399, -24.0434) centre (-8.0399, -24.0434) ccw
  arc A77 (-12.0399, -24.0434) -> (-11.747, -24.7505) centre (-11.0399, -24.0434) ccw
  line L190 (-7.3328, -24.7505) -> (-9.2399, -26.6576)
  line L191 (-11.747, -24.7505) -> (-9.8399, -26.6576)
  line L192 (-9.5399, -26.6576) -> (-9.2399, -26.6576)
  line L193 (-9.5399, -26.6576) -> (-9.8399, -26.6576)
  line L194 (-12.0399, -24.0434) -> (-12.0399, -7.2718)
  line L195 (-7.0399, -7.2718) -> (-7.0399, -24.0434)
  arc A78 (-11.747, -6.5647) -> (-12.0399, -7.2718) centre (-11.0399, -7.2718) ccw
  line L196 (-11.747, -6.5647) -> (-9.8399, -4.6576)
  line L197 (-9.5399, -4.6576) -> (-9.8399, -4.6576)
  line L198 (-9.5399, -4.6576) -> (-9.2399, -4.6576)
  arc A79 (-7.0399, -7.2718) -> (-7.3328, -6.5647) centre (-8.0399, -7.2718) ccw
  line L199 (-7.3328, -6.5647) -> (-9.2399, -4.6576)
  arc A80 (-31.0328, -30.2647) -> (-30.3257, -30.5576) centre (-30.3257, -29.5576) ccw
  arc A81 (-30.3257, -25.5576) -> (-31.0328, -25.8505) centre (-30.3257, -26.5576) ccw
  line L200 (-31.0328, -30.2647) -> (-32.9399, -28.3576)
  line L201 (-31.0328, -25.8505) -> (-32.9399, -27.7576)
  line L202 (-32.9399, -28.0576) -> (-32.9399, -28.3576)
  line L203 (-32.9399, -28.0576) -> (-32.9399, -27.7576)
  line L204 (-30.3257, -25.5576) -> (-13.5541, -25.5576)
  line L205 (-13.5541, -30.5576) -> (-30.3257, -30.5576)
  arc A82 (-12.847, -25.8505) -> (-13.5541, -25.5576) centre (-13.5541, -26.5576) ccw
  line L206 (-12.847, -25.8505) -> (-10.9399, -27.7576)
  line L207 (-10.9399, -28.0576) -> (-10.9399, -27.7576)
  line L208 (-10.9399, -28.0576) -> (-10.9399, -28.3576)
  arc A83 (-13.5541, -30.5576) -> (-12.847, -30.2647) centre (-13.5541, -29.5576) ccw
  line L209 (-12.847, -30.2647) -> (-10.9399, -28.3576)
  arc A84 (-77.8328, 19.3353) -> (-77.1257, 19.0424) centre (-77.1257, 20.0424) ccw
  arc A85 (-77.1257, 24.0424) -> (-77.8328, 23.7495) centre (-77.1257, 23.0424) ccw
  line L210 (-77.8328, 19.3353) -> (-79.7399, 21.2424)
  line L211 (-77.8328, 23.7495) -> (-79.7399, 21.8424)
  line L212 (-79.7399, 21.5424) -> (-79.7399, 21.2424)
  line L213 (-79.7399, 21.5424) -> (-79.7399, 21.8424)
  line L214 (-77.1257, 24.0424) -> (-60.3541, 24.0424)
  line L215 (-60.3541, 19.0424) -> (-77.1257, 19.0424)
  arc A86 (-59.647, 23.7495) -> (-60.3541, 24.0424) centre (-60.3541, 23.0424) ccw
  line L216 (-59.647, 23.7495) -> (-57.7399, 21.8424)
  line L217 (-57.7399, 21.5424) -> (-57.7399, 21.8424)
  line L218 (-57.7399, 21.5424) -> (-57.7399, 21.2424)
  arc A87 (-60.3541, 19.0424) -> (-59.647, 19.3353) centre (-60.3541, 20.0424) ccw
  line L219 (-59.647, 19.3353) -> (-57.7399, 21.2424)
  arc A88 (-77.8328, -5.4647) -> (-77.1257, -5.7576) centre (-77.1257, -4.7576) ccw
  arc A89 (-77.1257, -0.7576) -> (-77.8328, -1.0505) centre (-77.1257, -1.7576) ccw
  line L220 (-77.8328, -5.4647) -> (-79.7399, -3.5576)
  line L221 (-77.8328, -1.0505) -> (-79.7399, -2.9576)
  line L222 (-79.7399, -3.2576) -> (-79.7399, -3.5576)
  line L223 (-79.7399, -3.2576) -> (-79.7399, -2.9576)
  line L224 (-77.1257, -0.7576) -> (-60.3541, -0.7576)
  line L225 (-60.3541, -5.7576) -> (-77.1257, -5.7576)
  arc A90 (-59.647, -1.0505) -> (-60.3541, -0.7576) centre (-60.3541, -1.7576) ccw
  line L226 (-59.647, -1.0505) -> (-57.7399, -2.9576)
  line L227 (-57.7399, -3.2576) -> (-57.7399, -2.9576)
  line L228 (-57.7399, -3.2576) -> (-57.7399, -3.5576)
  arc A91 (-60.3541, -5.7576) -> (-59.647, -5.4647) centre (-60.3541, -4.7576) ccw
  line L229 (-59.647, -5.4647) -> (-57.7399, -3.5576)
  arc A92 (-78.9328, 0.0495) -> (-78.6399, 0.7566) centre (-79.6399, 0.7566) ccw
  arc A93 (-83.6399, 0.7566) -> (-83.347, 0.0495) centre (-82.6399, 0.7566) ccw
  line L230 (-78.9328, 0.0495) -> (-80.8399, -1.8576)
  line L231 (-83.347, 0.0495) -> (-81.4399, -1.8576)
  line L232 (-81.1399, -1.8576) -> (-80.8399, -1.8576)
  line L233 (-81.1399, -1.8576) -> (-81.4399, -1.8576)
  line L234 (-83.6399, 0.7566) -> (-83.6399, 17.5282)
  line L235 (-78.6399, 17.5282) -> (-78.6399, 0.7566)
  arc A94 (-83.347, 18.2353) -> (-83.6399, 17.5282) centre (-82.6399, 17.5282) ccw
  line L236 (-83.347, 18.2353) -> (-81.4399, 20.1424)
  line L237 (-81.1399, 20.1424) -> (-81.4399, 20.1424)
  line L238 (-81.1399, 20.1424) -> (-80.8399, 20.1424)
  arc A95 (-78.6399, 17.5282) -> (-78.9328, 18.2353) centre (-79.6399, 17.5282) ccw
  line L239 (-78.9328, 18.2353) -> (-80.8399, 20.1424)
  arc A96 (-78.9328, -24.7505) -> (-78.6399, -24.0434) centre (-79.6399, -24.0434) ccw
  arc A97 (-83.6399, -24.0434) -> (-83.347, -24.7505) centre (-82.6399, -24.0434) ccw
  line L240 (-78.9328, -24.7505) -> (-80.8399, -26.6576)
  line L241 (-83.347, -24.7505) -> (-81.4399, -26.6576)
  line L242 (-81.1399, -26.6576) -> (-80.8399, -26.6576)
  line L243 (-81.1399, -26.6576) -> (-81.4399, -26.6576)
  line L244 (-83.6399, -24.0434) -> (-83.6399, -7.2718)
  line L245 (-78.6399, -7.2718) -> (-78.6399, -24.0434)
  arc A98 (-83.347, -6.5647) -> (-83.6399, -7.2718) centre (-82.6399, -7.2718) ccw
  line L246 (-83.347, -6.5647) -> (-81.4399, -4.6576)
  line L247 (-81.1399, -4.6576) -> (-81.4399, -4.6576)
  line L248 (-81.1399, -4.6576) -> (-80.8399, -4.6576)
  arc A99 (-78.6399, -7.2718) -> (-78.9328, -6.5647) centre (-79.6399, -7.2718) ccw
  line L249 (-78.9328, -6.5647) -> (-80.8399, -4.6576)
  arc A100 (-54.1328, 0.0495) -> (-53.8399, 0.7566) centre (-54.8399, 0.7566) ccw
  arc A101 (-58.8399, 0.7566) -> (-58.547, 0.0495) centre (-57.8399, 0.7566) ccw
  line L250 (-54.1328, 0.0495) -> (-56.0399, -1.8576)
  line L251 (-58.547, 0.0495) -> (-56.6399, -1.8576)
  line L252 (-56.3399, -1.8576) -> (-56.0399, -1.8576)
  line L253 (-56.3399, -1.8576) -> (-56.6399, -1.8576)
  line L254 (-58.8399, 0.7566) -> (-58.8399, 17.5282)
  line L255 (-53.8399, 17.5282) -> (-53.8399, 0.7566)
  arc A102 (-58.547, 18.2353) -> (-58.8399, 17.5282) centre (-57.8399, 17.5282) ccw
  line L256 (-58.547, 18.2353) -> (-56.6399, 20.1424)
  line L257 (-56.3399, 20.1424) -> (-56.6399, 20.1424)
  line L258 (-56.3399, 20.1424) -> (-56.0399, 20.1424)
  arc A103 (-53.8399, 17.5282) -> (-54.1328, 18.2353) centre (-54.8399, 17.5282) ccw
  line L259 (-54.1328, 18.2353) -> (-56.0399, 20.1424)
  arc A104 (-54.1328, -24.7505) -> (-53.8399, -24.0434) centre (-54.8399, -24.0434) ccw
  arc A105 (-58.8399, -24.0434) -> (-58.547, -24.7505) centre (-57.8399, -24.0434) ccw
  line L260 (-54.1328, -24.7505) -> (-56.0399, -26.6576)
  line L261 (-58.547, -24.7505) -> (-56.6399, -26.6576)
  line L262 (-56.3399, -26.6576) -> (-56.0399, -26.6576)
  line L263 (-56.3399, -26.6576) -> (-56.6399, -26.6576)
  line L264 (-58.8399, -24.0434) -> (-58.8399, -7.2718)
  line L265 (-53.8399, -7.2718) -> (-53.8399, -24.0434)
  arc A106 (-58.547, -6.5647) -> (-58.8399, -7.2718) centre (-57.8399, -7.2718) ccw
  line L266 (-58.547, -6.5647) -> (-56.6399, -4.6576)
  line L267 (-56.3399, -4.6576) -> (-56.6399, -4.6576)
  line L268 (-56.3399, -4.6576) -> (-56.0399, -4.6576)
  arc A107 (-53.8399, -7.2718) -> (-54.1328, -6.5647) centre (-54.8399, -7.2718) ccw
  line L269 (-54.1328, -6.5647) -> (-56.0399, -4.6576)
  arc A108 (-77.8328, -30.2647) -> (-77.1257, -30.5576) centre (-77.1257, -29.5576) ccw
  arc A109 (-77.1257, -25.5576) -> (-77.8328, -25.8505) centre (-77.1257, -26.5576) ccw
  line L270 (-77.8328, -30.2647) -> (-79.7399, -28.3576)
  line L271 (-77.8328, -25.8505) -> (-79.7399, -27.7576)
  line L272 (-79.7399, -28.0576) -> (-79.7399, -28.3576)
  line L273 (-79.7399, -28.0576) -> (-79.7399, -27.7576)
  line L274 (-77.1257, -25.5576) -> (-60.3541, -25.5576)
  line L275 (-60.3541, -30.5576) -> (-77.1257, -30.5576)
  arc A110 (-59.647, -25.8505) -> (-60.3541, -25.5576) centre (-60.3541, -26.5576) ccw
  line L276 (-59.647, -25.8505) -> (-57.7399, -27.7576)
  line L277 (-57.7399, -28.0576) -> (-57.7399, -27.7576)
  line L278 (-57.7399, -28.0576) -> (-57.7399, -28.3576)
  arc A111 (-60.3541, -30.5576) -> (-59.647, -30.2647) centre (-60.3541, -29.5576) ccw
  line L279 (-59.647, -30.2647) -> (-57.7399, -28.3576)
  arc A112 (-115.1328, 19.3353) -> (-114.4257, 19.0424) centre (-114.4257, 20.0424) ccw
  arc A113 (-114.4257, 24.0424) -> (-115.1328, 23.7495) centre (-114.4257, 23.0424) ccw
  line L280 (-115.1328, 19.3353) -> (-117.0399, 21.2424)
  line L281 (-115.1328, 23.7495) -> (-117.0399, 21.8424)
  line L282 (-117.0399, 21.5424) -> (-117.0399, 21.2424)
  line L283 (-117.0399, 21.5424) -> (-117.0399, 21.8424)
  line L284 (-114.4257, 24.0424) -> (-97.6541, 24.0424)
  line L285 (-97.6541, 19.0424) -> (-114.4257, 19.0424)
  arc A114 (-96.947, 23.7495) -> (-97.6541, 24.0424) centre (-97.6541, 23.0424) ccw
  line L286 (-96.947, 23.7495) -> (-95.0399, 21.8424)
  line L287 (-95.0399, 21.5424) -> (-95.0399, 21.8424)
  line L288 (-95.0399, 21.5424) -> (-95.0399, 21.2424)
  arc A115 (-97.6541, 19.0424) -> (-96.947, 19.3353) centre (-97.6541, 20.0424) ccw
  line L289 (-96.947, 19.3353) -> (-95.0399, 21.2424)
  arc A116 (-115.1328, -5.4647) -> (-114.4257, -5.7576) centre (-114.4257, -4.7576) ccw
  arc A117 (-114.4257, -0.7576) -> (-115.1328, -1.0505) centre (-114.4257, -1.7576) ccw
  line L290 (-115.1328, -5.4647) -> (-117.0399, -3.5576)
  line L291 (-115.1328, -1.0505) -> (-117.0399, -2.9576)
  line L292 (-117.0399, -3.2576) -> (-117.0399, -3.5576)
  line L293 (-117.0399, -3.2576) -> (-117.0399, -2.9576)
  line L294 (-114.4257, -0.7576) -> (-97.6541, -0.7576)
  line L295 (-97.6541, -5.7576) -> (-114.4257, -5.7576)
  arc A118 (-96.947, -1.0505) -> (-97.6541, -0.7576) centre (-97.6541, -1.7576) ccw
  line L296 (-96.947, -1.0505) -> (-95.0399, -2.9576)
  line L297 (-95.0399, -3.2576) -> (-95.0399, -2.9576)
  line L298 (-95.0399, -3.2576) -> (-95.0399, -3.5576)
  arc A119 (-97.6541, -5.7576) -> (-96.947, -5.4647) centre (-97.6541, -4.7576) ccw
  line L299 (-96.947, -5.4647) -> (-95.0399, -3.5576)
  arc A120 (-116.2328, 0.0495) -> (-115.9399, 0.7566) centre (-116.9399, 0.7566) ccw
  arc A121 (-120.9399, 0.7566) -> (-120.647, 0.0495) centre (-119.9399, 0.7566) ccw
  line L300 (-116.2328, 0.0495) -> (-118.1399, -1.8576)
  line L301 (-120.647, 0.0495) -> (-118.7399, -1.8576)
  line L302 (-118.4399, -1.8576) -> (-118.1399, -1.8576)
  line L303 (-118.4399, -1.8576) -> (-118.7399, -1.8576)
  line L304 (-120.9399, 0.7566) -> (-120.9399, 17.5282)
  line L305 (-115.9399, 17.5282) -> (-115.9399, 0.7566)
  arc A122 (-120.647, 18.2353) -> (-120.9399, 17.5282) centre (-119.9399, 17.5282) ccw
  line L306 (-120.647, 18.2353) -> (-118.7399, 20.1424)
  line L307 (-118.4399, 20.1424) -> (-118.7399, 20.1424)
  line L308 (-118.4399, 20.1424) -> (-118.1399, 20.1424)
  arc A123 (-115.9399, 17.5282) -> (-116.2328, 18.2353) centre (-116.9399, 17.5282) ccw
  line L309 (-116.2328, 18.2353) -> (-118.1399, 20.1424)
  arc A124 (-116.2328, -24.7505) -> (-115.9399, -24.0434) centre (-116.9399, -24.0434) ccw
  arc A125 (-120.9399, -24.0434) -> (-120.647, -24.7505) centre (-119.9399, -24.0434) ccw
  line L310 (-116.2328, -24.7505) -> (-118.1399, -26.6576)
  line L311 (-120.647, -24.7505) -> (-118.7399, -26.6576)
  line L312 (-118.4399, -26.6576) -> (-118.1399, -26.6576)
  line L313 (-118.4399, -26.6576) -> (-118.7399, -26.6576)
  line L314 (-120.9399, -24.0434) -> (-120.9399, -7.2718)
  line L315 (-115.9399, -7.2718) -> (-115.9399, -24.0434)
  arc A126 (-120.647, -6.5647) -> (-120.9399, -7.2718) centre (-119.9399, -7.2718) ccw
  line L316 (-120.647, -6.5647) -> (-118.7399, -4.6576)
  line L317 (-118.4399, -4.6576) -> (-118.7399, -4.6576)
  line L318 (-118.4399, -4.6576) -> (-118.1399, -4.6576)
  arc A127 (-115.9399, -7.2718) -> (-116.2328, -6.5647) centre (-116.9399, -7.2718) ccw
  line L319 (-116.2328, -6.5647) -> (-118.1399, -4.6576)
  arc A128 (-91.4328, 0.0495) -> (-91.1399, 0.7566) centre (-92.1399, 0.7566) ccw
  arc A129 (-96.1399, 0.7566) -> (-95.847, 0.0495) centre (-95.1399, 0.7566) ccw
  line L320 (-91.4328, 0.0495) -> (-93.3399, -1.8576)
  line L321 (-95.847, 0.0495) -> (-93.9399, -1.8576)
  line L322 (-93.6399, -1.8576) -> (-93.3399, -1.8576)
  line L323 (-93.6399, -1.8576) -> (-93.9399, -1.8576)
  line L324 (-96.1399, 0.7566) -> (-96.1399, 17.5282)
  line L325 (-91.1399, 17.5282) -> (-91.1399, 0.7566)
  arc A130 (-95.847, 18.2353) -> (-96.1399, 17.5282) centre (-95.1399, 17.5282) ccw
  line L326 (-95.847, 18.2353) -> (-93.9399, 20.1424)
  line L327 (-93.6399, 20.1424) -> (-93.9399, 20.1424)
  line L328 (-93.6399, 20.1424) -> (-93.3399, 20.1424)
  arc A131 (-91.1399, 17.5282) -> (-91.4328, 18.2353) centre (-92.1399, 17.5282) ccw
  line L329 (-91.4328, 18.2353) -> (-93.3399, 20.1424)
  arc A132 (-91.4328, -24.7505) -> (-91.1399, -24.0434) centre (-92.1399, -24.0434) ccw
  arc A133 (-96.1399, -24.0434) -> (-95.847, -24.7505) centre (-95.1399, -24.0434) ccw
  line L330 (-91.4328, -24.7505) -> (-93.3399, -26.6576)
  line L331 (-95.847, -24.7505) -> (-93.9399, -26.6576)
  line L332 (-93.6399, -26.6576) -> (-93.3399, -26.6576)
  line L333 (-93.6399, -26.6576) -> (-93.9399, -26.6576)
  line L334 (-96.1399, -24.0434) -> (-96.1399, -7.2718)
  line L335 (-91.1399, -7.2718) -> (-91.1399, -24.0434)
  arc A134 (-95.847, -6.5647) -> (-96.1399, -7.2718) centre (-95.1399, -7.2718) ccw
  line L336 (-95.847, -6.5647) -> (-93.9399, -4.6576)
  line L337 (-93.6399, -4.6576) -> (-93.9399, -4.6576)
  line L338 (-93.6399, -4.6576) -> (-93.3399, -4.6576)
  arc A135 (-91.1399, -7.2718) -> (-91.4328, -6.5647) centre (-92.1399, -7.2718) ccw
  line L339 (-91.4328, -6.5647) -> (-93.3399, -4.6576)
  arc A136 (-115.1328, -30.2647) -> (-114.4257, -30.5576) centre (-114.4257, -29.5576) ccw
  arc A137 (-114.4257, -25.5576) -> (-115.1328, -25.8505) centre (-114.4257, -26.5576) ccw
  line L340 (-115.1328, -30.2647) -> (-117.0399, -28.3576)
  line L341 (-115.1328, -25.8505) -> (-117.0399, -27.7576)
  line L342 (-117.0399, -28.0576) -> (-117.0399, -28.3576)
  line L343 (-117.0399, -28.0576) -> (-117.0399, -27.7576)
  line L344 (-114.4257, -25.5576) -> (-97.6541, -25.5576)
  line L345 (-97.6541, -30.5576) -> (-114.4257, -30.5576)
  arc A138 (-96.947, -25.8505) -> (-97.6541, -25.5576) centre (-97.6541, -26.5576) ccw
  line L346 (-96.947, -25.8505) -> (-95.0399, -27.7576)
  line L347 (-95.0399, -28.0576) -> (-95.0399, -27.7576)
  line L348 (-95.0399, -28.0576) -> (-95.0399, -28.3576)
  arc A139 (-97.6541, -30.5576) -> (-96.947, -30.2647) centre (-97.6541, -29.5576) ccw
  line L349 (-96.947, -30.2647) -> (-95.0399, -28.3576)
  arc A140 (90.3672, 19.3353) -> (91.0743, 19.0424) centre (91.0743, 20.0424) ccw
  arc A141 (91.0743, 24.0424) -> (90.3672, 23.7495) centre (91.0743, 23.0424) ccw
  line L350 (90.3672, 19.3353) -> (88.4601, 21.2424)
  line L351 (90.3672, 23.7495) -> (88.4601, 21.8424)
  line L352 (88.4601, 21.5424) -> (88.4601, 21.2424)
  line L353 (88.4601, 21.5424) -> (88.4601, 21.8424)
  line L354 (91.0743, 24.0424) -> (107.8459, 24.0424)
  line L355 (107.8459, 19.0424) -> (91.0743, 19.0424)
  arc A142 (108.553, 23.7495) -> (107.8459, 24.0424) centre (107.8459, 23.0424) ccw
  line L356 (108.553, 23.7495) -> (110.4601, 21.8424)
  line L357 (110.4601, 21.5424) -> (110.4601, 21.8424)
  line L358 (110.4601, 21.5424) -> (110.4601, 21.2424)
  arc A143 (107.8459, 19.0424) -> (108.553, 19.3353) centre (107.8459, 20.0424) ccw
  line L359 (108.553, 19.3353) -> (110.4601, 21.2424)
  arc A144 (90.3672, -5.4647) -> (91.0743, -5.7576) centre (91.0743, -4.7576) ccw
  arc A145 (91.0743, -0.7576) -> (90.3672, -1.0505) centre (91.0743, -1.7576) ccw
  line L360 (90.3672, -5.4647) -> (88.4601, -3.5576)
  line L361 (90.3672, -1.0505) -> (88.4601, -2.9576)
  line L362 (88.4601, -3.2576) -> (88.4601, -3.5576)
  line L363 (88.4601, -3.2576) -> (88.4601, -2.9576)
  line L364 (91.0743, -0.7576) -> (107.8459, -0.7576)
  line L365 (107.8459, -5.7576) -> (91.0743, -5.7576)
  arc A146 (108.553, -1.0505) -> (107.8459, -0.7576) centre (107.8459, -1.7576) ccw
  line L366 (108.553, -1.0505) -> (110.4601, -2.9576)
  line L367 (110.4601, -3.2576) -> (110.4601, -2.9576)
  line L368 (110.4601, -3.2576) -> (110.4601, -3.5576)
  arc A147 (107.8459, -5.7576) -> (108.553, -5.4647) centre (107.8459, -4.7576) ccw
  line L369 (108.553, -5.4647) -> (110.4601, -3.5576)
  arc A148 (89.2672, 0.0495) -> (89.5601, 0.7566) centre (88.5601, 0.7566) ccw
  arc A149 (84.5601, 0.7566) -> (84.853, 0.0495) centre (85.5601, 0.7566) ccw
  line L370 (89.2672, 0.0495) -> (87.3601, -1.8576)
  line L371 (84.853, 0.0495) -> (86.7601, -1.8576)
  line L372 (87.0601, -1.8576) -> (87.3601, -1.8576)
  line L373 (87.0601, -1.8576) -> (86.7601, -1.8576)
  line L374 (84.5601, 0.7566) -> (84.5601, 17.5282)
  line L375 (89.5601, 17.5282) -> (89.5601, 0.7566)
  arc A150 (84.853, 18.2353) -> (84.5601, 17.5282) centre (85.5601, 17.5282) ccw
  line L376 (84.853, 18.2353) -> (86.7601, 20.1424)
  line L377 (87.0601, 20.1424) -> (86.7601, 20.1424)
  line L378 (87.0601, 20.1424) -> (87.3601, 20.1424)
  arc A151 (89.5601, 17.5282) -> (89.2672, 18.2353) centre (88.5601, 17.5282) ccw
  line L379 (89.2672, 18.2353) -> (87.3601, 20.1424)
  arc A152 (89.2672, -24.7505) -> (89.5601, -24.0434) centre (88.5601, -24.0434) ccw
  arc A153 (84.5601, -24.0434) -> (84.853, -24.7505) centre (85.5601, -24.0434) ccw
  line L380 (89.2672, -24.7505) -> (87.3601, -26.6576)
  line L381 (84.853, -24.7505) -> (86.7601, -26.6576)
  line L382 (87.0601, -26.6576) -> (87.3601, -26.6576)